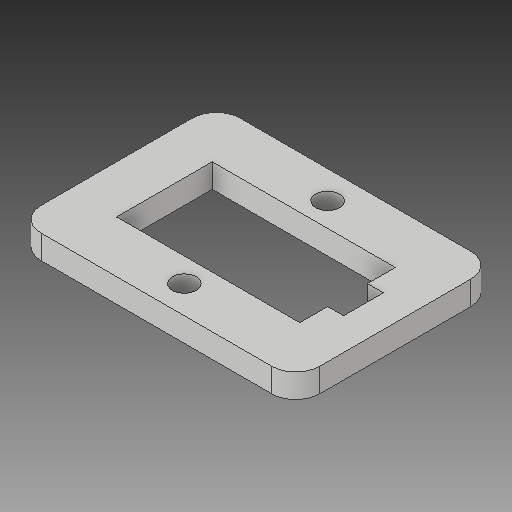
# Autodesk Inventor part: 板子4
Saved by Autodesk Inventor 2017 (Build 210142000, 142)
## iProperties
Part Number: 板子4
Material: 一般
Document SubType Name: Modeling
Designer: User
Density: 1 g/cm^3
Appearance: 預設
Author: User
Autodesk Inventor part; units mm, degrees
ref_plane "YZ Plane" through (0, 0, 0) normal (1, 0, 0) x (0, 1, 0)
ref_plane "XZ Plane" through (0, 0, 0) normal (0, 1, 0) x (-1, 0, 0)
ref_plane "XY Plane" through (0, 0, 0) normal (0, 0, 1) x (1, 0, 0)
sketch "草圖1" plane through (0, 0, 0) normal (0, 1, 0) x (-1, 0, 0)
  line L0 (17.5, 12.5) -> (-17.5, 12.5)
  line L1 (-17.5, 12.5) -> (-17.5, -12.5)
  line L2 (-17.5, -12.5) -> (17.5, -12.5)
  line L3 (17.5, -12.5) -> (17.5, 12.5)
  line L4 (24.5, 0) -> (-24.5, 0) projected
  line L5 (0, -17.5) -> (0, 17.5) projected
  circle A0 centre (0, 9) radius 1.5
  line L6 (11.5, 0) -> (-11.5, 0)
  line L7 (-11.5, 0) -> (-11.5, 6)
  line L8 (-11.5, 6) -> (11.5, 6)
  line L9 (11.5, 6) -> (11.5, 0)
  line L10 (-11.5, 0) -> (-13.5, 0)
  line L11 (-13.5, 0) -> (-13.5, 2.5)
  line L12 (-13.5, 2.5) -> (-11.5, 2.5)
  line L13 (-11.5, 2.5) -> (-11.5, 0)
  circle A1 centre (0, -9) radius 1.5
  line L14 (-11.5, 0) -> (-11.5, -6)
  line L15 (-11.5, -6) -> (11.5, -6)
  line L16 (11.5, -6) -> (11.5, 0)
  line L17 (-13.5, 0) -> (-13.5, -2.5)
  line L18 (-13.5, -2.5) -> (-11.5, -2.5)
  line L19 (-11.5, -2.5) -> (-11.5, 0)
  dimension "d103" = 25
  dimension "d104" = 35
  dimension "d105" = 17.5
  dimension "d106" = 12.5
  dimension "d107" = 3
  dimension "d109" = 6
  dimension "d110" = 6
  dimension "d111" = 23
  dimension "d112" = 2
  dimension "d113" = 2.5
  dimension "d115" = 18
  constraints: 36 end point, 6 parallel, 5 symmetric about line, 3 horizontal, 3 perpendicular, 2 centre point, 2 point on line, 1 other
  measures "d103" distance of L2.end L0.start
  measures "d104" distance of L0.start L0.end
  measures "d105" distance between parallel lines of L5 L3
  measures "d106" distance between parallel lines of L4 L2
  measures "d107" diameter of A0
  measures "d109" distance of L8.end L6.start
  measures "d110" distance between parallel lines of L3 L9
  measures "d111" distance of L7.end L8.end
  measures "d112" distance of L11.end L12.end
  measures "d113" distance of L10.end L11.end
  measures "d115" distance of A1.centre A0.centre
extrude "擠出2" add sketch "草圖1" along normal mid plane 3 contours L3 L4 L9 L8 L5 A0 L0 | L5 A0 L8 L7 L12 L11 L4 L1 L0 | L3 L2 L5 A1 L15 L16 L4 | L4 L17 L18 L14 L15 L5 A1 L2 L1
fillet "圓角2" radius 3 4 edges at (-17.5, 0, 12.5) (17.5, 0, 12.5) (17.5, 0, -12.5) (-17.5, 0, -12.5)
